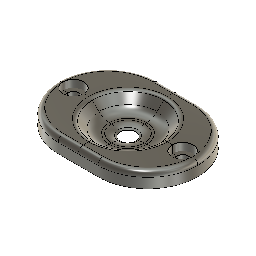
main_button_protector (Autodesk Fusion 360 design; units mm, degrees)
Autodesk Fusion 360 part; units mm, degrees
note: some values were not read from the file. Chosen so that the rebuilt part matches the saved one: which face or edge a step refers to; which pieces of a blend or face edit are solid. Set by a fixed rule: which sketch regions a step uses.
sketch "Skizze1" plane through (0, 0, 0) normal (0, 0, 1) x (1, 0, 0)
  line L0 (0, 0) -> (14, 0)
  line L1 (14, 0) -> (14, 10)
  line L2 (14, 10) -> (0, 10)
  line L3 (0, 10) -> (0, 0)
  dimension "d1" = 14
  dimension "d2" = 10
  constraint horizontal L0
  constraint vertical L1
  constraint horizontal L2
  constraint vertical L3
  constraint coincident L0.start L3.end
  measures "d1" distance of L0.start L0.end
  measures "d2" distance of L0.end L1.end
extrude "Extrusion1" add sketch "Skizze1" along normal blind 3 makes body 1
sketch "Skizze2" plane through (0, 0, 3) normal (0, 0, 1) x (-1, 0, 0)
  line L0 (0, -10) -> (0, 0)
  line L1 (0, 0) -> (-14, 0)
  line L2 (-14, 0) -> (-14, -10)
  line L3 (-14, -10) -> (0, -10)
  constraint coincident L0.end L1.start
hole "Bohrung1" at (0, 0, 3) direction (0, 0, -1) diameter 3.2 depth 18 tip angle 180 bodies 1
sketch "Skizze3" plane through (0, 0, 3) normal (0, 0, 1) x (-1, 0, 0)
  arc A0 (-1.6, 0) -> (0, -1.6) centre (0, 0) ccw
  line L0 (-1.6, 0) -> (-14, 0)
  line L1 (-14, 0) -> (-14, -10)
  line L2 (-14, -10) -> (0, -10)
  line L3 (0, -10) -> (0, -1.6)
  circle A1 centre (0, 0) radius 5
  dimension "d8" = 10
  constraint concentric A0 A1
  measures "d8" diameter of A1
extrude "Extrusion2" cut sketch "Skizze3" against normal blind 2.5 contours A0 L0 L3 A1 | A0 L0 L3 A1 bodies 1
chamfer "Fase1" distance 0.5 distance2 1 1 edges at (1.1314, 1.1314, 0.5) measured on face at (1.5928, 0.1521, 0.1667) on bodies 1
chamfer "Fase2" distance 2.5 distance2 2.5 1 edges at (3.5355, 3.5355, 3) measured on face at (10.8494, 4.0257, 3) on bodies 1
sketch "Skizze4" plane through (0, 0, 3) normal (0, 0, 1) x (-1, 0, 0)
  line L0 (-7.5, 0) -> (-14, 0)
  line L1 (-14, 0) -> (-14, -10)
  line L2 (-14, -10) -> (0, -10)
  line L3 (0, -10) -> (0, -7.5)
  arc A0 (-7.5, 0) -> (0, -7.5) centre (0, 0) ccw
  point P0 (-11, 0)
  dimension "d15" = 3
  constraint coincident L0 P0
  measures "d15" distance of L1 P0
hole "Bohrung2" at (11, 0, 3) direction (0, 0, -1) diameter 2.4 end through all counterbore diameter 4.2 counterbore depth 1.5 bodies 1
fillet "Abrundung1" radius 10 1 edges at (14, 10, 1.5) on bodies 1
fillet "Abrundung2" radius 3 3 edges at (3.5355, 3.5355, 0.5005) (3.5355, 3.5355, 0.5) (1.8383, 1.8383, 0.5) on bodies 1
fillet "Abrundung3" radius 1 3 edges at (5.3033, 5.3033, 3) (11.0711, 7.0711, 3) (2, 10, 3) on bodies 1
mirror "Spiegeln1" about plane through (0, 0, 0) normal (0, -1, 0) of "Extrusion1", "Extrusion2", "Fase1", "Fase2", "Bohrung2", "Abrundung1", "Abrundung2", "Abrundung3" makes body 2
mirror "Spiegeln2" about plane through (0, -10, 0) normal (-1, 0, 0) of "Extrusion1", "Extrusion2", "Fase1", "Fase2", "Bohrung2", "Abrundung1", "Abrundung2", "Abrundung3", "Spiegeln1" makes body 3 at (-6.5033, 3.5458, 0) makes body 4 at (-6.5033, -3.5458, 0)
